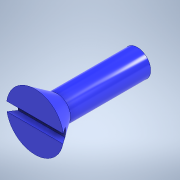
# Autodesk Inventor part: Pieza7_tornillo
Saved by Autodesk Inventor 2021 (Build 250183000, 183)
## iProperties
Created: 2020-10-13
Part Number: Pieza7_tornillo
Material: Iron, Cast
Document SubType Name: Modeling
Designer: ENRIQUE
Density: 7.15 g/cm^3
Appearance: Blue - Wall Paint - Glossy
Author: ENRIQUE
Autodesk Inventor part; units mm, degrees
ref_plane "YZ Plane" through (0, 0, 0) normal (1, 0, 0) x (0, 1, 0)
ref_plane "XZ Plane" through (0, 0, 0) normal (0, 1, 0) x (-1, 0, 0)
ref_plane "XY Plane" through (0, 0, 0) normal (0, 0, 1) x (1, 0, 0)
sketch "Sketch3" plane through (0, 0, 0) normal (0, 0, 1) x (1, 0, 0)
  circle A0 centre (0, 0) radius 3
  dimension "d9" = 6
  constraints: 1 centre point, 1 coincident
  measures "d9" diameter of A0
extrude "Extrusion1" add sketch "Sketch3" against normal blind 18
sketch "Sketch4" plane through (0, 0, 0) normal (1, 0, 0) x (0, 1, 0)
  line L0 (-3, -18) -> (3, -18) projected
  line L1 (0, -19.7321) -> (3, -18)
  line L2 (0, -18) -> (0, -19.7321)
  point P0 (0, 0)
  constraints: 4 end point, 1 midpoint, 1 vertical
revolve "Revolution1" add sketch "Sketch4" angle 360 mid plane about axis through (0, 0, -18) along (0, 0, -1)
sketch "Sketch5" plane through (0, 0, 0) normal (0, 1, 0) x (-1, 0, 0)
  line L0 (3, 0) -> (-3, 0) projected
  line L1 (3, 0) -> (6.385, 5)
  line L2 (6.385, 5) -> (0, 5)
  line L3 (0, 5) -> (0, 0)
  dimension "d14" = 5
  dimension "d15" = 6.385
  constraints: 6 end point, 1 horizontal, 1 perpendicular
  measures "d14" vertical distance of L0.start L1.end
  measures "d15" distance of L1.end L2.end
revolve "Revolution2" add sketch "Sketch5" angle 360 about axis through (0, 0, 5) along (0, 0, -1)
sketch "Sketch6" plane through (0, 0, 0) normal (1, 0, 0) x (0, 1, 0)
  line L0 (-6.385, 5) -> (6.385, 5) projected
  line L1 (-1.15, 5) -> (-1.15, 3.5)
  line L2 (-1.15, 3.5) -> (-0.15, 3.5)
  line L3 (-0.15, 3.5) -> (0.85, 3.5)
  line L4 (0.85, 3.5) -> (0.85, 5)
  point P0 (0, 0)
  dimension "d17" = 1
  dimension "d18" = 1.5
  constraints: 8 end point, 3 perpendicular, 3 point on line, 1 collinear
  measures "d17" distance of L1.end L2.end
  measures "d18" distance of L3.end L4.end
extrude "Extrusion2" cut sketch "Sketch6" along normal mid plane 20
body "Solid1"
